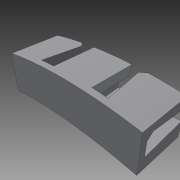
# Autodesk Inventor part: HanesBand-Adjuster
Saved by Autodesk Inventor 2015 (Build 190159000, 159)
## iProperties
Created: 2020-03-26
Part Number: HanesBand-Adjuster
Material: Generic
Document SubType Name: Modeling
Designer: Dominick Lee
Density: 1 g/cm^3
Appearance: Default
Author: Dominick Lee
Autodesk Inventor part; units mm, degrees
ref_plane "YZ Plane" through (0, 0, 0) normal (1, 0, 0) x (0, 1, 0)
ref_plane "XZ Plane" through (0, 0, 0) normal (0, 1, 0) x (-1, 0, 0)
ref_plane "XY Plane" through (0, 0, 0) normal (0, 0, 1) x (1, 0, 0)
sketch "Sketch1" plane through (0, 0, 0) normal (0, 1, 0) x (-1, 0, 0)
  line L0 (12.5, 3) -> (-12.5, 3)
  line L1 (-12.5, 3) -> (-12.5, -3)
  line L2 (-12.5, -3) -> (12.5, -3)
  line L3 (12.5, -3) -> (12.5, 3)
  line L4 (12.5, 3) -> (-12.5, -3) construction
  line L5 (-12.5, 3) -> (12.5, -3) construction
  line L6 (0, -3) -> (0, -4)
  arc A0 (12.5, -4) -> (-12.5, -4) centre (0, -81.625) ccw
  line L7 (12.5, -4) -> (12.5, -3)
  line L8 (-12.5, -4) -> (-12.5, -3)
  line L9 (0, 3) -> (0, 4)
  arc A1 (12.5, 3) -> (-12.5, 3) centre (0, -74.625) ccw
  point P0 (0, 0)
  dimension "d0" = 25
  dimension "d1" = 6
  dimension "d47" = 1
  dimension "d48" = 1
  constraints: 20 end point, 6 point on circle, 4 midpoint, 4 vertical, 2 centre point, 2 parallel, 1 horizontal, 1 perpendicular
  measures "d0" distance of L0.start L0.end
  measures "d1" distance of L1.end L0.end
  measures "d47" distance of L6.start L6.end
  measures "d48" distance of L9.start L9.end
extrude "Extrusion1" add sketch "Sketch1" along normal blind 1.2
sketch "Sketch2" plane through (0, 1.2, 0) normal (0, 1, 0) x (1, 0, 0)
  line L0 (12.5, -3) -> (12.5, -1.8)
  line L1 (-12.5, -1.8) -> (-12.5, -3)
  line L2 (-12.5, -2.4) -> (-6.5, -2.4)
  line L3 (12.5, -2.4) -> (6.5, -2.4)
  line L4 (-6.5, -1.8) -> (-6.5, -3)
  line L5 (6.5, -1.8) -> (6.5, -3)
  line L6 (-6.5, -1.8) -> (-12.5, -1.8)
  line L7 (12.5, -1.8) -> (6.5, -1.8)
  line L8 (-12.5, -3) -> (-6.5, -3)
  line L9 (6.5, -3) -> (12.5, -3)
  line L10 (-1.5, -1.8) -> (-1.5, 1.8)
  line L11 (-1.5, 1.8) -> (1.5, 1.8)
  line L12 (1.5, 1.8) -> (1.5, -1.8)
  line L13 (-1.5, -1.8) -> (1.5, 1.8) construction
  line L14 (-1.5, 1.8) -> (1.5, -1.8) construction
  line L15 (12.5, 1.8) -> (1.5, 1.8)
  line L16 (-1.5, 1.8) -> (-12.5, 1.8)
  line L17 (-3.3159, -1.8) -> (-1.5, -1.8)
  line L18 (1.5, -1.8) -> (3.3274, -1.8)
  arc A0 (-12.5, 4) -> (12.5, 4) centre (0, 81.625) ccw
  arc A1 (-12.5, -3) -> (12.5, -3) centre (0, 74.625) ccw
  arc A2 (-12.5, -3) -> (12.5, -3) centre (0, 74.625) ccw projected
  line L19 (-6.5, -3) -> (-6.4892, -3.7318)
  line L20 (6.5, -3) -> (6.5, -3.7309)
  line L21 (6.5, -3) -> (7.2309, -3) construction
  line L22 (3.7, -3) -> (4.6129, -3) construction
  line L23 (-12.5, 4) -> (-12.5, 1.8)
  line L24 (12.5, 4) -> (12.5, 1.8)
  line L25 (-6.4892, -3.7318) -> (-6.1486, -1.8)
  line L26 (-6.4892, -3.7318) -> (-4.5277, -3.7318) construction
  line L27 (-6.1486, -1.8) -> (-6.5, -1.8)
  line L28 (-3.6885, -3.9134) -> (-3.3159, -1.8)
  line L29 (-3.6885, -3.9134) -> (-1.5425, -3.9134) construction
  line L30 (3.7, -3.9129) -> (3.3274, -1.8)
  line L31 (3.7, -3.9129) -> (5.8455, -3.9129) construction
  line L32 (6.5, -3.7309) -> (6.1595, -1.8)
  line L33 (6.5, -3.7309) -> (8.4606, -3.7309) construction
  line L34 (6.1595, -1.8) -> (6.5, -1.8)
  point P0 (0, 0)
  dimension "d14" = 1.2
  dimension "d34" = 6
  dimension "d36" = 6
  dimension "d43" = 3
  dimension "d49" = 90
  dimension "d51" = 80
  dimension "d52" = 80
  dimension "d53" = 100
  dimension "d54" = 100
  constraints: 70 end point, 14 horizontal, 10 point on circle, 6 parallel, 5 equal length, 4 vertical, 3 perpendicular, 2 centre point, 2 midpoint
  measures "d14" distance of L0.end L0.start
  measures "d34" distance of L2.start L2.end
  measures "d36" distance of L3.start L3.end
  measures "d43" distance of L10.end L11.end
  measures "d49" angle of L20 L21
  measures "d51" angle of L26 L25
  measures "d52" angle of L29 L28
  measures "d53" angle of L31 L30
  measures "d54" angle of L33 L32
extrude "Extrusion3" add sketch "Sketch2" along normal blind 8
draft "FaceDraft1" angle 5 pull direction (0, -1, 0) faces at (5.1667, 3.8667, -1.8) (-8.8333, 3.8667, -1.8) fixed edges at (-7, 1.2, -1.8) (7, 1.2, -1.8)
draft "FaceDraft2" angle 5 pull direction (0, -1, 0) faces at (10.3865, 3.8667, 1.8) fixed edges at (9.3298, 1.2, 1.8)
draft "FaceDraft4" angle 2.5 pull direction (0, -1, 0) faces at (-8.2657, 3.8667, 1.8) fixed edges at (-9.3243, 1.2, 1.8)
chamfer "Chamfer3" distance 1.8 angle 45 2 edges at (-1.5, 5.2, 1.8) (1.5, 5.2, 1.8)
draft "FaceDraft9" angle -8 pull direction (0, 1, 0) faces at (-6.2416, 6.5333, 2.3275) fixed edges at (-6.3189, 1.2, 2.7659)
draft "FaceDraft10" angle -8 pull direction (0, 1, 0) faces at (6.2319, 6.5333, 2.2103) fixed edges at (6.3298, 1.2, 2.7654)
chamfer "Chamfer4" distance 1 angle 45 2 edges at (-5.1539, 9.2, 2.6338) (5.1339, 9.2, 2.4581)
chamfer "Chamfer5" distance 1 angle 45 2 edges at (9.3298, 1.2, 1.8) (-9.3243, 1.2, 1.8)
body "Solid1"
